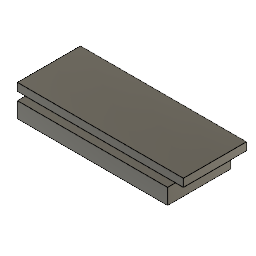
incubetter wire cover (Autodesk Fusion 360 design; units mm, degrees)
Autodesk Fusion 360 part; units mm, degrees
sketch "Sketch1" plane through (0, 0, 0) normal (0, 0, 1) x (1, 0, 0)
  line L0 (9.5, 4) -> (-9.5, 4)
  line L1 (-9.5, 4) -> (-9.5, -4)
  line L2 (-9.5, -4) -> (9.5, -4)
  line L3 (9.5, -4) -> (9.5, 4)
  line L4 (9.5, 4) -> (-9.5, -4) construction
  line L5 (-9.5, 4) -> (9.5, -4) construction
  dimension "d1" = 19
  dimension "d2" = 8
extrude "Extrude1" add sketch "Sketch1" along normal blind 2
sketch "Sketch2" plane through (0, 0, 2) normal (0, 0, 1) x (-1, 0, 0)
  line L0 (-9.5, 4) -> (-9.5, -4)
  line L1 (-9.5, -4) -> (9.5, -4)
  line L2 (9.5, -4) -> (9.5, 4)
  line L3 (9.5, 4) -> (-9.5, 4)
  line L4 (0, 4) -> (0, 3)
  line L5 (0, 3) -> (0, -5)
  line L6 (-10.5, -5) -> (10.5, -5)
  line L7 (10.5, -5) -> (10.5, 3)
  line L8 (10.5, 3) -> (-10.5, 3)
  line L9 (-10.5, 3) -> (-10.5, -5)
  line L10 (-10.5, -5) -> (10.5, 3) construction
  line L11 (10.5, -5) -> (-10.5, 3) construction
  dimension "d5" = 21
extrude "Extrude2" add sketch "Sketch2" along normal blind 1 contours L0 L1 L5 L8 | L0 L1 L5 L6 L8 L9 | L1 L2 L5 L8 | L1 L2 L5 L6 L7 L8
